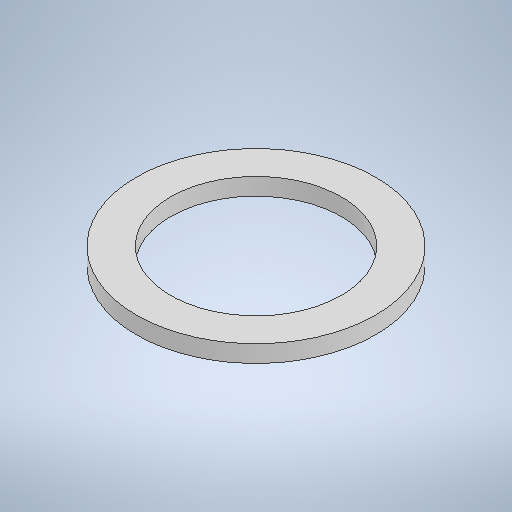
# Autodesk Inventor part: Bearing_Belt_Distance_Sleeve
Saved by Autodesk Inventor 2025.1 (Build 291241020, 241B)
## iProperties
Created: 2024-11-07
Part Number: Bearing_Belt_Distance_Sleeve
Material: Generic
Document SubType Name: Modeling
Designer: leon-
Density: 1 g/cm^3
Appearance: Default
Author: leon-
Autodesk Inventor part; units mm, degrees
ref_plane "YZ Plane" through (0, 0, 0) normal (1, 0, 0) x (0, 1, 0)
ref_plane "XZ Plane" through (0, 0, 0) normal (0, 1, 0) x (-1, 0, 0)
ref_plane "XY Plane" through (0, 0, 0) normal (0, 0, 1) x (1, 0, 0)
sketch "Sketch1" plane through (0, 0, 0) normal (0, 1, 0) x (-1, 0, 0)
  circle A0 centre (0, 0) radius 2.5
  circle A1 centre (0, 0) radius 3.5
  dimension "d0" = 5
  dimension "d1" = 7
  constraints: 2 centre point, 2 coincident
  measures "d0" diameter of A0
  measures "d1" diameter of A1
extrude "Extrusion1" add sketch "Sketch1" along normal blind 0.5
body "Solid1"
